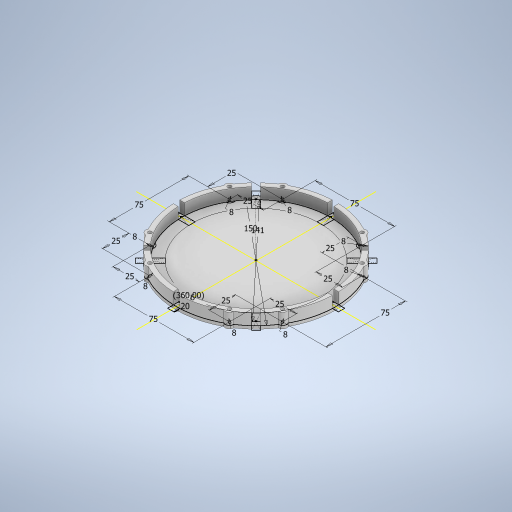
# Autodesk Inventor part: board_holder
Saved by Autodesk Inventor 2024.3 (Build 283343000, 343)
## iProperties
Created: 2026-05-02
Part Number: board_holder
Material: Generic
Document SubType Name: Modeling
Designer: owozn
Density: 1 g/cm^3
Appearance: Default
Author: owozn
Autodesk Inventor part; units mm, degrees
ref_plane "YZ Plane" through (0, 0, 0) normal (1, 0, 0) x (0, 1, 0)
ref_plane "XZ Plane" through (0, 0, 0) normal (0, 1, 0) x (-1, 0, 0)
ref_plane "XY Plane" through (0, 0, 0) normal (0, 0, 1) x (1, 0, 0)
sketch "Sketch1" plane through (0, 0, 0) normal (0, 1, 0) x (-1, 0, 0)
  line L0 (0, -112.7) -> (0, 112.7) projected
  line L1 (112.7, 0) -> (-112.7, 0) projected
  circle A0 centre (0, 0) radius 70.5
  circle A1 centre (0, 0) radius 75
  line L2 (3, 80.5) -> (-3, 80.5)
  line L3 (-3, 80.5) -> (-3, 60.5)
  line L4 (-3, 60.5) -> (3, 60.5)
  line L5 (3, 60.5) -> (3, 80.5)
  line L6 (3, 80.5) -> (-3, 60.5) construction
  line L7 (-3, 80.5) -> (3, 60.5) construction
  line L8 (-40.6586, 44.9013) -> (-54.8008, 59.0434)
  line L9 (-54.8008, 59.0434) -> (-59.0434, 54.8008)
  line L10 (-59.0434, 54.8008) -> (-44.9013, 40.6586)
  line L11 (-59.0434, 54.8008) -> (-40.6586, 44.9013) construction
  line L12 (-54.8008, 59.0434) -> (-44.9013, 40.6586) construction
  line L13 (-44.9013, 40.6586) -> (-40.6586, 44.9013)
  line L14 (-60.5, 3) -> (-80.5, 3)
  line L15 (-80.5, 3) -> (-80.5, -3)
  line L16 (-80.5, -3) -> (-60.5, -3)
  line L17 (-80.5, -3) -> (-60.5, 3) construction
  line L18 (-80.5, 3) -> (-60.5, -3) construction
  line L19 (-60.5, -3) -> (-60.5, 3)
  line L20 (-44.9013, -40.6586) -> (-59.0434, -54.8008)
  line L21 (-59.0434, -54.8008) -> (-54.8008, -59.0434)
  line L22 (-54.8008, -59.0434) -> (-40.6586, -44.9013)
  line L23 (-54.8008, -59.0434) -> (-44.9013, -40.6586) construction
  line L24 (-59.0434, -54.8008) -> (-40.6586, -44.9013) construction
  line L25 (-40.6586, -44.9013) -> (-44.9013, -40.6586)
  line L26 (-3, -60.5) -> (-3, -80.5)
  line L27 (-3, -80.5) -> (3, -80.5)
  line L28 (3, -80.5) -> (3, -60.5)
  line L29 (3, -80.5) -> (-3, -60.5) construction
  line L30 (-3, -80.5) -> (3, -60.5) construction
  line L31 (3, -60.5) -> (-3, -60.5)
  line L32 (40.6586, -44.9013) -> (54.8008, -59.0434)
  line L33 (54.8008, -59.0434) -> (59.0434, -54.8008)
  line L34 (59.0434, -54.8008) -> (44.9013, -40.6586)
  line L35 (59.0434, -54.8008) -> (40.6586, -44.9013) construction
  line L36 (54.8008, -59.0434) -> (44.9013, -40.6586) construction
  line L37 (44.9013, -40.6586) -> (40.6586, -44.9013)
  line L38 (60.5, -3) -> (80.5, -3)
  line L39 (80.5, -3) -> (80.5, 3)
  line L40 (80.5, 3) -> (60.5, 3)
  line L41 (80.5, 3) -> (60.5, -3) construction
  line L42 (80.5, -3) -> (60.5, 3) construction
  line L43 (60.5, 3) -> (60.5, -3)
  line L44 (44.9013, 40.6586) -> (59.0434, 54.8008)
  line L45 (59.0434, 54.8008) -> (54.8008, 59.0434)
  line L46 (54.8008, 59.0434) -> (40.6586, 44.9013)
  line L47 (54.8008, 59.0434) -> (44.9013, 40.6586) construction
  line L48 (59.0434, 54.8008) -> (40.6586, 44.9013) construction
  line L49 (40.6586, 44.9013) -> (44.9013, 40.6586)
  line L50 (49.851, -49.851) -> (0, 0) construction
  circle A2 centre (-62.5, -37.5) radius 4
  circle A3 centre (-62.5, 37.5) radius 4
  circle A4 centre (-37.5, 62.5) radius 4
  circle A5 centre (37.5, 62.5) radius 4
  circle A6 centre (62.5, 37.5) radius 4
  circle A7 centre (62.5, -37.5) radius 4
  circle A8 centre (37.5, -62.5) radius 4
  circle A9 centre (-37.5, -62.5) radius 4
  point P0 (0, 70.5)
  point P1 (-49.851, 49.851)
  point P2 (-70.5, 0)
  point P3 (-49.851, -49.851)
  point P4 (0, -70.5)
  point P5 (49.851, -49.851)
  point P6 (70.5, 0)
  point P7 (49.851, 49.851)
  point P8 (55.1119, 50.8692)
  point P9 (51.9272, 47.6846)
  point P10 (70.4361, 3)
  point P11 (74.94, 3)
  point P12 (47.6846, 51.9272)
  point P13 (50.8692, 55.1119)
  point P14 (3, 74.94)
  point P15 (3, 70.4361)
  point P16 (-50.8692, 55.1119)
  point P17 (-47.6846, 51.9272)
  point P18 (-3, 70.4361)
  point P19 (-3, 74.94)
  point P20 (-74.94, 3)
  point P21 (-70.4361, 3)
  point P22 (-51.9272, 47.6846)
  point P23 (-55.1119, 50.8692)
  point P24 (-55.1119, -50.8692)
  point P25 (-51.9272, -47.6846)
  point P26 (-70.4361, -3)
  point P27 (-74.94, -3)
  point P28 (-3, -74.94)
  point P29 (-3, -70.4361)
  point P30 (-47.6846, -51.9272)
  point P31 (-50.8692, -55.1119)
  point P32 (50.8692, -55.1119)
  point P33 (47.6846, -51.9272)
  point P34 (3, -70.4361)
  point P35 (3, -74.94)
  point P36 (74.94, -3)
  point P37 (70.4361, -3)
  point P38 (51.9272, -47.6846)
  point P39 (55.1119, -50.8692)
  point P40 (-62.4721, -41.4999)
  point P41 (-66.0162, -35.593)
  point P42 (-35.593, -66.0162)
  point P43 (-41.4999, -62.4721)
  point P44 (41.4999, -62.4721)
  point P45 (35.593, -66.0162)
  point P46 (66.0162, -35.593)
  point P47 (62.4721, -41.4999)
  point P48 (62.4721, 41.4999)
  point P49 (66.0162, 35.593)
  point P50 (35.593, 66.0162)
  point P51 (41.4999, 62.4721)
  point P52 (-41.4999, 62.4721)
  point P53 (-35.593, 66.0162)
  point P54 (-62.4721, 41.4999)
  point P55 (-66.0162, 35.593)
  dimension "d0" = 141
  dimension "d1" = 150
  dimension "d4" = 6
  dimension "d5" = 20
  dimension "d8" = 360
  dimension "d14" = 25
  dimension "d16" = 25
  dimension "d21" = 75
  dimension "d22" = 25
  dimension "d23" = 25
  dimension "d24" = 25
  dimension "d25" = 25
  dimension "d26" = 75
  dimension "d27" = 25
  dimension "d28" = 25
  dimension "d29" = 75
  dimension "d30" = 75
  dimension "d31" = 8
  dimension "d32" = 8
  dimension "d33" = 8
  dimension "d34" = 8
  dimension "d35" = 8
  dimension "d36" = 8
  dimension "d37" = 8
  dimension "d38" = 8
  constraints: 98 end point, 10 coincident, 8 centre point, 3 midpoint, 3 parallel, 2 symmetric about line, 1 horizontal, 1 horizontal alignment, 1 perpendicular, 1 point on line, 94 other
  measures "d4" distance of L4.end L3.end
  measures "d5" distance of L3.end L2.end
  measures "d14" horizontal distance of point (62.5, -37.5) point (37.5, -62.5)
  measures "d16" horizontal distance of point (62.5, -37.5) point (37.5, -62.5)
  measures "d21" distance of point (-37.5, -62.5) point (37.5, -62.5)
  measures "d22" horizontal distance of point (-37.5, 62.5) point (-62.5, 37.5)
  measures "d23" horizontal distance of point (-37.5, 62.5) point (-62.5, 37.5)
  measures "d24" horizontal distance of point (62.5, 37.5) point (37.5, 62.5)
  measures "d25" horizontal distance of point (37.5, 62.5) point (62.5, 37.5)
  measures "d26" distance of point (62.5, 37.5) point (62.5, -37.5)
  measures "d27" horizontal distance of point (-62.5, -37.5) point (-37.5, -62.5)
  measures "d28" horizontal distance of point (-62.5, -37.5) point (-37.5, -62.5)
  measures "d29" distance of point (-62.5, -37.5) point (-62.5, 37.5)
  measures "d30" distance of point (37.5, 62.5) point (-37.5, 62.5)
  measures "d31" diameter of A2
  measures "d32" diameter of A3
  measures "d33" diameter of A4
  measures "d34" diameter of A5
  measures "d35" diameter of A6
  measures "d36" diameter of A7
  measures "d37" diameter of A8
  measures "d38" diameter of A9
extrude "Extrusion2" add sketch "Sketch1" against normal blind 3 contours A1 L26 A0 L0 | L0 A0 L28 A1 | A0 L26 L31 L0 | L0 L31 L28 A0 | A1 A9 A0 L26 | L28 A0 A8 A1 | L31 L26 A0 A9 L22 L25 L20 A2 L16 L19 L1 L0 | L0 L1 L43 L38 A0 A7 L34 L37 L32 A8 L28 L31 | A9 A1 | A1 A9 A0 | A8 A0 A1 | A1 A8 | L1 L19 L14 A0 A3 L10 L13 L8 A4 L3 L4 L0 | L0 L4 L5 A0 A5 L46 L49 L44 A6 L40 L43 L1 | A0 A9 | A8 A0 | A1 L22 A0 A9 | A8 A0 L32 A1 | L4 L3 A0 L0 | L0 A0 L5 L4 | L43 L40 A0 L1 | L1 A0 L38 L43 | L19 L16 A0 L1 | L1 A0 L14 L19 | A1 L20 A0 L22 | L32 A0 L34 A1 | A0 L3 A1 L0 | L0 A1 L5 A0 | A0 L40 A1 L1 | L1 A1 L38 A0 | A0 L16 A1 L1 | L1 A1 L14 A0 | A0 L20 L25 L22 | L32 L37 L34 A0 | A1 A2 A0 L20 | L34 A0 A7 A1 | L5 A1 A5 A0 | A0 A4 A1 L3 | A0 A6 A1 L40 | L38 A1 A7 A0 | L14 A1 A3 A0 | A0 A2 A1 L16 | A2 A1 | A1 A2 A0 | A7 A0 A1 | A1 A7 | A5 A1 A0 | A0 A5 | A4 A0 | A0 A4 A1 | A6 A0 | A0 A6 A1 | A0 A7 | A3 A1 A0 | A0 A3 | A2 A0 | A5 A1 | A1 A4 | A5 A1 L46 A0 | A0 L8 A1 A4 | A1 A6 | A0 L44 A1 A6 | A3 A1 | A3 A1 L10 A0 | L46 A1 L44 A0 | A0 L44 L49 L46 | L8 L13 L10 A0 | A0 L10 A1 L8
extrude "Extrusion3" add sketch "Sketch1" along normal blind 10.5 contours A1 A9 A0 L26 | L28 A0 A8 A1 | A9 A1 | A1 A9 A0 | A8 A0 A1 | A1 A8 | A1 L22 A0 A9 | A8 A0 L32 A1 | A1 A2 A0 L20 | L34 A0 A7 A1 | L5 A1 A5 A0 | A0 A4 A1 L3 | A0 A6 A1 L40 | L38 A1 A7 A0 | L14 A1 A3 A0 | A0 A2 A1 L16 | A2 A1 | A1 A2 A0 | A7 A0 A1 | A1 A7 | A5 A1 A0 | A0 A4 A1 | A0 A6 A1 | A3 A1 A0 | A5 A1 | A1 A4 | A5 A1 L46 A0 | A0 L8 A1 A4 | A1 A6 | A0 L44 A1 A6 | A3 A1 | A3 A1 L10 A0
hole "Hole1" at (-37.5, 0, -62.5) at (37.5, 0, -62.5) at (62.5, 0, -37.5) at (62.5, 0, 37.5) at (37.5, 0, 62.5) at (-37.5, 0, 62.5) at (-62.5, 0, 37.5) at (-62.5, 0, -37.5) direction (0, -1, 0) diameter 3.5 end through all both
body "Solid1"
